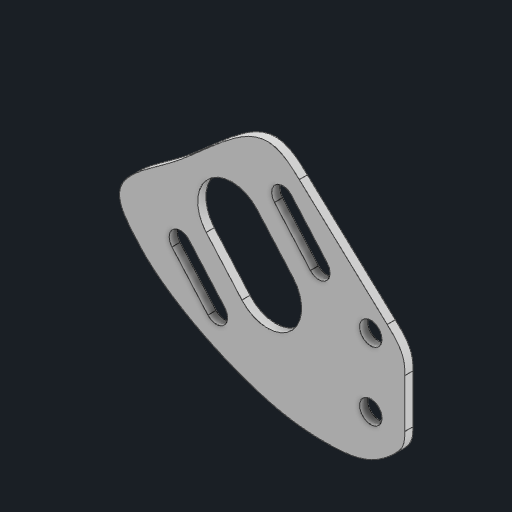
# Autodesk Inventor part: third-stage
Saved by Autodesk Inventor 2023.2 (Build 272271000, 271)
## iProperties
Created: 2023-03-29
Part Number: third-stage
Material: Generic
Document SubType Name: Modeling
Designer: Liam
Density: 1 g/cm^3
Appearance: Default
Author: Liam
Autodesk Inventor part; units mm, degrees
ref_plane "YZ Plane" through (0, 0, 0) normal (1, 0, 0) x (0, 1, 0)
ref_plane "XZ Plane" through (0, 0, 0) normal (0, 1, 0) x (-1, 0, 0)
ref_plane "XY Plane" through (0, 0, 0) normal (0, 0, 1) x (1, 0, 0)
sketch "Sketch1" plane through (0, 0, 0) normal (0, 0, 1) x (1, 0, 0)
  line L0 (-72.8164, 47.6422) -> (-79.5151, 55.2811)
  line L1 (-63.5697, 69.2654) -> (-56.8709, 61.6266)
  circle A0 centre (-45.6184, 44.45) radius 2.0955
  circle A1 centre (-45.6184, 57.15) radius 2.0955
  line L2 (-78.2217, 69.8899) -> (-79.1765, 69.0525)
  line L3 (-88.4889, 49.5267) -> (-89.3263, 50.4816)
  spline S0 degree 4 poles (-89.3263, 50.4816) (-91.643, 53.1234) (-96.2764, 58.4071) (-85.3251, 63.6606) (-81.226, 67.2552) (-79.1765, 69.0525) knots 0 0 0 0 0 0.5 1 1 1 1 1
  line L4 (-78.2217, 69.8899) -> (-77.2668, 70.7272)
  line L5 (-58.947, 75.2527) -> (-42.5605, 60.0661)
  line L6 (-88.4889, 49.5267) -> (-86.4935, 47.2513) construction
  line L7 (-86.4935, 47.2513) -> (-79.1765, 41.658) construction
  line L8 (-79.1765, 41.658) -> (-65.6397, 36.2801) construction
  line L9 (-65.6397, 36.2801) -> (-57.5295, 35.1145) construction
  line L10 (-57.5295, 35.1145) -> (-50.9347, 35.1145) construction
  line L11 (-50.9347, 35.1145) -> (-45.158, 36.0858) construction
  line L12 (-45.158, 36.0858) -> (-41.2186, 39.8714) construction
  spline S1 degree 4 poles (-88.4889, 49.5267) (-86.4935, 47.2513) (-79.1765, 41.658) (-65.6397, 36.2801) (-57.5295, 35.1145) (-50.9347, 35.1145) (-45.158, 36.0858) (-41.2186, 39.8714) knots 1 1 1 1 1 2 3 4 5 5 5 5 5
  line L13 (-39.2684, 44.45) -> (-39.2684, 53.473)
  spline S2 degree 4 poles (-39.2684, 53.473) (-39.2684, 54.4427) (-39.2684, 56.382) (-40.4685, 58.1273) (-41.8632, 59.4198) (-42.5605, 60.0661) knots 0 0 0 0 0 0.5 1 1 1 1 1
  spline S3 degree 4 poles (-39.2684, 44.45) (-39.2684, 43.803) (-39.2684, 42.5091) (-39.8191, 41.2162) (-40.7521, 40.3196) (-41.2186, 39.8714) knots 0 0 0 0 0 0.5 1 1 1 1 1
  spline S4 degree 4 poles (-77.2668, 70.7272) (-75.394, 72.3695) (-71.6485, 75.6541) (-65.3075, 81.1475) (-61.0671, 77.2177) (-58.947, 75.2527) knots 0 0 0 0 0 0.5 1 1 1 1 1
  line L14 (-60.0895, 58.8441) -> (-66.7486, 66.4377)
  line L15 (-69.638, 50.4706) -> (-76.2972, 58.0643)
  line L16 (-53.7199, 64.3898) -> (-60.4186, 72.0287)
  line L17 (-75.9674, 44.879) -> (-82.6661, 52.5179)
  arc A2 (-75.9674, 44.879) -> (-72.8164, 47.6422) centre (-74.3919, 46.2606) ccw
  arc A3 (-79.5151, 55.2811) -> (-82.6661, 52.5179) centre (-81.0906, 53.8995) ccw
  arc A4 (-56.8709, 61.6266) -> (-53.7199, 64.3898) centre (-55.2954, 63.0082) ccw
  arc A5 (-60.4186, 72.0287) -> (-63.5697, 69.2654) centre (-61.9942, 70.647) ccw
  arc A6 (-69.638, 50.4706) -> (-60.0895, 58.8441) centre (-64.8638, 54.6573) ccw
  arc A7 (-66.7486, 66.4377) -> (-76.2972, 58.0643) centre (-71.5229, 62.251) ccw
  line L18 (-82.6661, 52.5179) -> (-79.5151, 55.2811) construction
  line L19 (-76.2972, 58.0643) -> (-66.7486, 66.4377) construction
  line L20 (-63.5697, 69.2654) -> (-60.4186, 72.0287) construction
  point P0 (0, 0)
  point P1 (-79.3931, 52.0233)
  point P2 (-61.9743, 70.6245)
  point P3 (-81.0715, 53.8776)
  point P4 (-71.5229, 62.251)
  point P5 (-81.0906, 53.8995)
  dimension "d18" = 1.27
  dimension "d20" = 1.27
  dimension "d22" = 1.27
  dimension "d23" = 4.191
  dimension "d24" = 4.191
  dimension "d42" = 10.16
  dimension "d43" = 10.16
  dimension "d47" = 4.191
  dimension "d48" = 4.191
  dimension "d51" = 6.35
  dimension "d52" = 6.35
  dimension "d54" = 12.7
  dimension "d55" = 12.7
  dimension "d56" = 12.7
  dimension "d57" = 12.7
  constraints: 28 end point, 12 point on circle, 8 centre point, 8 parallel, 7 tangent, 3 midpoint, 2 perpendicular, 2 point on line, 2 vertical, 1 horizontal, 20 other
  measures "d18" distance of L2.start L2.end
  measures "d20" distance of L3.start L3.end
  measures "d22" distance of L2.start L4.end
  measures "d23" diameter of A0
  measures "d24" diameter of A1
  measures "d42" distance of L0.start L0.end
  measures "d43" distance of L1.start L1.end
  measures "d47" distance between parallel lines of L0 L17
  measures "d48" distance between parallel lines of L16 L1
  measures "d51" radius of A6
  measures "d52" radius of A7
  measures "d54" distance of point (-71.523, 62.251) point (-61.994, 70.647)
  measures "d55" distance of point (-81.091, 53.899) A7.centre
  measures "d56" distance of A6.centre A4.centre
  measures "d57" distance of A2.centre A6.centre
extrude "Extrusion3" add sketch "Sketch1" along normal blind 1.524
body "Solid3"
